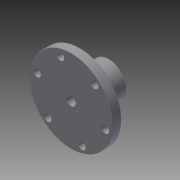
# Autodesk Inventor part: 6 mm Set Hub
Saved by Autodesk Inventor 2014 (Build 180170000, 170)
## iProperties
Created: 2015-10-07
Part Number: 6 mm Set Hub
Material: Generisch
Document SubType Name: Modeling
Designer: nrk
Density: 1 g/cm^3
Appearance: Vorgabe
Author: nrk
Autodesk Inventor part; units mm, degrees
ref_plane "XZ Plane" through (0, 0, 0) normal (0, 1, 0) x (-1, 0, 0)
ref_plane "XY Plane" through (0, 0, 0) normal (0, 0, 1) x (1, 0, 0)
sketch "Skizze1" plane through (0, 0, 0) normal (0, 1, 0) x (-1, 0, 0)
  circle A0 centre (0, 0) radius 28.5
  dimension "d0" = 57
  constraints: 1 centre point, 1 coincident
  measures "d0" diameter of A0
extrude "Extrusion1" add sketch "Skizze1" along normal blind 6
sketch "Skizze2" plane through (0, 6, 0) normal (0, 1, 0) x (1, 0, 0)
  circle A0 centre (0, 0) radius 28.5 projected
  circle A1 centre (-16.0851, 17.8121) radius 2.5
  circle A2 centre (0, 0) radius 24 construction
  dimension "d4" = 48
  dimension "d3" = 5
  constraints: 1 centre point, 1 coincident, 3 other
  measures "d3" diameter of A1
extrude "Extrusion2" cut sketch "Skizze2" against normal through all contours A1
pattern_circular "Runde Anordnung1" count 6 over 360 about axis through (0, -10, 0) along (0, 1, 0) of "Extrusion2"
sketch "Skizze3" plane through (0, 6, 0) normal (0, 1, 0) x (1, 0, 0)
  circle A0 centre (0, 0) radius 28.5 projected
  circle A1 centre (0, 0) radius 12
  dimension "d10" = 24
  constraints: 1 centre point, 1 coincident
  measures "d10" diameter of A1
extrude "Extrusion3" add sketch "Skizze3" along normal blind 20 contours A1
sketch "Skizze4" plane through (0, 26, 0) normal (0, 1, 0) x (1, 0, 0)
  circle A0 centre (0, 0) radius 12 projected
  circle A1 centre (0, 0) radius 3
  dimension "d13" = 6
  constraints: 1 centre point, 1 coincident
  measures "d13" diameter of A1
extrude "Extrusion4" cut sketch "Skizze4" against normal through all contours A1
fillet "Rundung1" radius 0.25 1 edges at (-6.1332, 0, 25.0012)
fillet "Rundung2" radius 0.25 1 edges at (18.5851, 0, 17.8121)
fillet "Rundung3" radius 0.25 1 edges at (24.7183, 0, -7.1891)
fillet "Rundung4" radius 0.25 1 edges at (6.1332, 0, -25.0012)
fillet "Rundung5" radius 0.25 1 edges at (-18.5851, 0, -17.8121)
fillet "Rundung6" radius 0.25 1 edges at (-24.7183, 0, 7.1891)
fillet "Rundung7" radius 0.25 1 edges at (-3, 0, 0)
fillet "Rundung8" radius 0.25 1 edges at (-18.5851, 6, -17.8121)
fillet "Rundung9" radius 0.25 1 edges at (6.1332, 6, -25.0012)
fillet "Rundung10" radius 0.25 1 edges at (24.7183, 6, -7.1891)
fillet "Rundung11" radius 0.25 1 edges at (18.5851, 6, 17.8121)
fillet "Rundung12" radius 0.25 1 edges at (-6.1332, 6, 25.0012)
fillet "Rundung13" radius 0.25 1 edges at (-24.7183, 6, 7.1891)
fillet "Rundung14" radius 0.25 1 edges at (28.5, 6, 0)
fillet "Rundung15" radius 0.25 1 edges at (-3, 26, 0)
fillet "Rundung16" radius 0.25 1 edges at (-12, 26, 0)
fillet "Rundung17" radius 0.25 1 edges at (28.5, 0, 0)
ref_plane "Arbeitsebene1" through (12, 0, 0) normal (1, 0, 0) x (0, 1, 0)
sketch "Skizze7" plane through (12, 0, 0) normal (1, 0, 0) x (0, 1, 0)
  line L0 (0, 0) -> (31.8146, 0) construction
  line L1 (0, 0) -> (0, 15.4066) construction
  line L2 (26, 11.75) -> (26, -11.75) projected
  point P0 (16, 0)
  dimension "d35" = 10
  constraints: 4 end point, 1 horizontal, 1 perpendicular, 1 point on line
  measures "d35" distance from line of point (16, 0) L2
hole "Bohrung1" at (12, 16, 0) direction (-1, 0, 0) diameter 4.134 end up to face face through (0, 26, 0) facing (0, -1, 0) round with radius 3 far side yes thread size "M5x0.8" class "6H" standard "ISO Metric profile"
